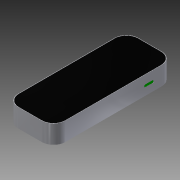
# Autodesk Inventor part: leapmotioncontroller
Saved by Autodesk Inventor 2015 (Build 190159000, 159)
## iProperties
Created: 2015-05-22
Part Number: leapmotioncontroller
Material: Generic
Document SubType Name: Modeling
Designer: Andrew
Density: 1 g/cm^3
Appearance: Default
Author: Andrew
Autodesk Inventor part; units mm, degrees
ref_plane "YZ Plane" through (0, 0, 0) normal (1, 0, 0) x (0, 1, 0)
ref_plane "XZ Plane" through (0, 0, 0) normal (0, 1, 0) x (-1, 0, 0)
ref_plane "XY Plane" through (0, 0, 0) normal (0, 0, 1) x (1, 0, 0)
sketch "Sketch1" plane through (0, 0, 0) normal (0, 1, 0) x (-1, 0, 0)
  line L0 (7.9375, 0) -> (23.8125, 0)
  line L1 (31.75, -7.9375) -> (31.75, -73.025)
  line L2 (23.8125, -80.9625) -> (7.9375, -80.9625)
  line L3 (0, -73.025) -> (0, -7.9375)
  arc A0 (31.75, -7.9375) -> (23.8125, 0) centre (23.8125, -7.9375) ccw
  arc A1 (23.8125, -80.9625) -> (31.75, -73.025) centre (23.8125, -73.025) ccw
  arc A2 (0, -73.025) -> (7.9375, -80.9625) centre (7.9375, -73.025) ccw
  arc A3 (7.9375, 0) -> (0, -7.9375) centre (7.9375, -7.9375) ccw
  point P0 (0, 0)
  point P1 (31.75, -80.9625)
  point P2 (31.75, 0)
  point P3 (0, -80.9625)
  dimension "d0" = 80.9625
  dimension "d1" = 31.75
  dimension "d2" = 7.9375
  dimension "d3" = 7.9375
  dimension "d4" = 7.9375
  dimension "d5" = 7.9375
  constraints: 8 end point, 8 point on circle, 8 point on line, 8 tangent, 4 centre point, 2 parallel, 1 horizontal, 1 perpendicular
  measures "d0" distance of point (31.75, 0) point (31.75, -80.962)
  measures "d1" distance of point (31.75, -80.962) point (0, -80.962)
  measures "d2" radius of A0
  measures "d3" radius of A1
  measures "d4" radius of A2
  measures "d5" radius of A3
extrude "Extrusion1" add sketch "Sketch1" along normal blind 12.446
sketch "Sketch2" plane through (0, 12.446, 0) normal (0, 1, 0) x (1, 0, 0)
  line L0 (-31.75, 73.025) -> (-31.75, 7.9375) projected
  line L1 (-31.75, 3.952) -> (-31.496, 3.952)
  line L2 (-23.8125, 0) -> (-7.9375, 0) projected
  line L3 (-15.875, 0) -> (-15.875, 0.254)
  line L4 (-7.9375, 80.9625) -> (-23.8125, 80.9625) projected
  line L5 (-15.875, 80.9625) -> (-15.875, 80.7085)
  line L6 (0, 7.9375) -> (0, 73.025) projected
  line L7 (0, 40.4812) -> (-0.254, 40.4812)
  line L8 (-23.5585, 0.254) -> (-8.1915, 0.254)
  line L9 (-0.254, 8.1915) -> (-0.254, 72.771)
  line L10 (-8.1915, 80.7085) -> (-23.5585, 80.7085)
  line L11 (-31.496, 72.771) -> (-31.496, 8.1915)
  arc A0 (-0.254, 72.771) -> (-8.1915, 80.7085) centre (-8.1915, 72.771) ccw
  arc A1 (-23.5585, 80.7085) -> (-31.496, 72.771) centre (-23.5585, 72.771) ccw
  arc A2 (-8.1915, 0.254) -> (-0.254, 8.1915) centre (-8.1915, 8.1915) ccw
  arc A3 (-31.496, 8.1915) -> (-23.5585, 0.254) centre (-23.5585, 8.1915) ccw
  point P0 (0, 0)
  dimension "d8" = 0.254
  dimension "d9" = 0.254
  dimension "d10" = 0.254
  dimension "d11" = 0.254
  dimension "d12" = 7.9375
  constraints: 16 end point, 8 point on circle, 8 tangent, 4 centre point, 3 equal radius, 3 midpoint, 2 horizontal, 2 parallel, 2 perpendicular, 2 vertical, 1 point on line
  measures "d8" distance of L1.start L1.end
  measures "d9" distance of L3.start L3.end
  measures "d10" distance of L5.start L5.end
  measures "d11" distance of L7.start L7.end
  measures "d12" radius of A0
extrude "Extrusion2" cut sketch "Sketch2" against normal blind 0.1016
sketch "Sketch3" plane through (-31.75, 0, -73.025) normal (-1, 0, 0) x (0, 0, 1)
  line L0 (65.0875, 0) -> (0, 0) projected
  line L1 (59.5609, 0) -> (59.5609, 5.08)
  line L2 (65.0875, 12.446) -> (65.0875, 6.604)
  line L3 (65.0875, 0) -> (65.0875, 12.446) projected
  line L4 (58.7672, 5.08) -> (54.0047, 5.08)
  line L5 (53.2109, 5.8737) -> (53.2109, 5.8737)
  line L6 (54.0047, 6.6675) -> (58.7672, 6.6675)
  line L7 (59.5609, 5.8737) -> (59.5609, 5.8737)
  arc A0 (54.0047, 6.6675) -> (53.2109, 5.8737) centre (54.0047, 5.8738) ccw
  arc A1 (53.2109, 5.8737) -> (54.0047, 5.08) centre (54.0047, 5.8737) ccw
  arc A2 (59.5609, 5.8737) -> (58.7672, 6.6675) centre (58.7672, 5.8738) ccw
  arc A3 (58.7672, 5.08) -> (59.5609, 5.8737) centre (58.7672, 5.8737) ccw
  point P0 (73.025, 0)
  point P1 (53.2109, 6.6675)
  point P2 (59.5609, 6.6675)
  dimension "d15" = 5.08
  dimension "d17" = 5.842
  dimension "d18" = 6.35
  dimension "d19" = 1.5875
  dimension "d20" = 0.7937
  constraints: 12 end point, 8 point on circle, 8 point on line, 8 tangent, 4 centre point, 3 equal radius, 2 parallel, 2 perpendicular, 1 horizontal
  measures "d15" distance of L1.start L1.end
  measures "d17" distance of L2.start L2.end
  measures "d18" distance of point (53.211, 6.667) point (59.561, 6.667)
  measures "d19" distance of point (59.561, 6.667) L1.end
  measures "d20" radius of A0
extrude "Extrusion3" cut sketch "Sketch3" against normal blind 0.0254
sketch "Sketch4" plane through (0, 0, 0) normal (0, -1, 0) x (1, 0, 0)
  line L0 (-23.5585, -0.254) -> (-8.1915, -0.254)
  line L1 (-0.254, -8.1915) -> (-0.254, -72.771)
  line L2 (-8.1915, -80.7085) -> (-23.5585, -80.7085)
  line L3 (-31.496, -72.771) -> (-31.496, -8.1915)
  arc A0 (-31.496, -72.771) -> (-23.5585, -80.7085) centre (-23.5585, -72.771) ccw
  arc A1 (-8.1915, -80.7085) -> (-0.254, -72.771) centre (-8.1915, -72.771) ccw
  arc A2 (-23.5585, -0.254) -> (-31.496, -8.1915) centre (-23.5585, -8.1915) ccw
  arc A3 (-0.254, -8.1915) -> (-8.1915, -0.254) centre (-8.1915, -8.1915) ccw
  point P0 (0, 0)
  dimension "d23" = 7.9375
  dimension "d24" = 7.9375
  dimension "d25" = 7.9375
  dimension "d26" = 7.9375
  constraints: 8 end point, 8 point on circle, 8 tangent, 4 centre point, 2 parallel, 1 horizontal, 1 perpendicular
  measures "d23" radius of A0
  measures "d24" radius of A1
  measures "d25" radius of A2
  measures "d26" radius of A3
extrude "Extrusion4" add sketch "Sketch4" along normal blind 0.0508
body "Solid1"
